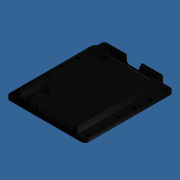
# Autodesk Inventor part: (45-0005) SpartanPi Base Housing
Saved by Autodesk Inventor 2015 (Build 190159000, 159)
## iProperties
Created: 2016-09-21
Part Number: (45-0005) SpartanPi Base Housing
Material: Generic
Document SubType Name: Modeling
Designer: Justin
Density: 1 g/cm^3
Appearance: Smooth - Black
Author: Justin
Autodesk Inventor part; units mm, degrees
ref_plane "YZ Plane" through (0, 0, 0) normal (1, 0, 0) x (0, 1, 0)
ref_plane "XZ Plane" through (0, 0, 0) normal (0, 1, 0) x (-1, 0, 0)
ref_plane "XY Plane" through (0, 0, 0) normal (0, 0, 1) x (1, 0, 0)
sketch "Sketch1" plane through (0, 0, 0) normal (0, 0, 1) x (1, 0, 0)
  line L0 (0, 0) -> (61, 0)
  line L1 (61, 0) -> (61, 90)
  line L2 (61, 90) -> (0, 90)
  line L3 (0, 90) -> (0, 0)
  dimension "d0" = 61
  dimension "d1" = 90
  constraints: 8 end point, 2 parallel, 1 horizontal, 1 perpendicular
  measures "d0" distance of L1.end L2.end
  measures "d1" distance of L0.end L1.end
extrude "Extrusion1" add sketch "Sketch1" along normal blind 10
fillet "Fillet1" radius 3 4 edges at (61, 90, 5) (0, 90, 5) (0, 0, 5) (61, 0, 5)
shell "Shell1" thickness 2 removed faces 1 at (40.6667, 31, 10)
sketch "Sketch8" plane through (0, 0, 10) normal (0, 0, 1) x (1, 0, 0)
  arc A0 (2, 3) -> (3, 2) centre (3, 3) ccw projected
  line L0 (2, 3) -> (2, 87) projected
  arc A1 (3, 88) -> (2, 87) centre (3, 87) ccw projected
  line L1 (3, 88) -> (58, 88) projected
  arc A2 (59, 87) -> (58, 88) centre (58, 87) ccw projected
  line L2 (59, 87) -> (59, 3) projected
  arc A3 (58, 2) -> (59, 3) centre (58, 3) ccw projected
  line L3 (58, 2) -> (3, 2) projected
  line L4 (58, 89.05) -> (3, 89.05)
  arc A4 (3, 89.05) -> (0.95, 87) centre (3, 87) ccw
  line L5 (0.95, 87) -> (0.95, 3)
  arc A5 (0.95, 3) -> (3, 0.95) centre (3, 3) ccw
  line L6 (3, 0.95) -> (58, 0.95)
  arc A6 (58, 0.95) -> (60.05, 3) centre (58, 3) ccw
  line L7 (60.05, 3) -> (60.05, 87)
  arc A7 (60.05, 87) -> (58, 89.05) centre (58, 87) ccw
  point P0 (0, 0)
  dimension "d59" = 1.05
  constraints: 8 end point, 8 point on circle, 4 centre point, 7 other
  measures "d59" distance between parallel lines of L4 L1
extrude "Extrusion8" cut sketch "Sketch8" against normal blind 1.05
sketch "Sketch2" plane through (3, 88, 2) normal (0, 0, 1) x (1, 0, 0)
  line L0 (56, -85) -> (56, -1) projected
  line L1 (55, 0) -> (0, 0) projected
  circle A0 centre (52, -4) radius 3
  circle A1 centre (52, -62) radius 3
  circle A2 centre (3, -4) radius 3
  circle A3 centre (3, -62) radius 3
  point P0 (-3, -88)
  dimension "d6" = 6
  dimension "d7" = 4
  dimension "d8" = 4
  dimension "d11" = 58
  dimension "d14" = 49
  constraints: 4 centre point, 1 horizontal, 1 vertical, 6 other
  measures "d6" diameter of A0
  measures "d7" distance from line of L1 A0.centre
  measures "d8" distance from line of L0 A0.centre
  measures "d11" distance of A0.centre A1.centre
  measures "d14" distance of A0.centre A2.centre
extrude "Extrusion2" add sketch "Sketch2" along normal blind 4
sketch "Sketch3" plane through (6, 26, 6) normal (0, 0, 1) x (1, 0, 0)
  circle A0 centre (0, 0) radius 3 projected
  circle A1 centre (49, 0) radius 3 projected
  circle A2 centre (49, 58) radius 3 projected
  circle A3 centre (0, 58) radius 3 projected
  circle A4 centre (49, 58) radius 1.125
  circle A5 centre (49, 0) radius 1.125
  circle A6 centre (0, 0) radius 1.125
  circle A7 centre (0, 58) radius 1.125
  point P0 (-6, -26)
  dimension "d19" = 2.25
  dimension "d20" = 2.25
  dimension "d21" = 2.25
  dimension "d22" = 2.25
  constraints: 4 centre point, 4 coincident
  measures "d19" diameter of A4
  measures "d20" diameter of A5
  measures "d21" diameter of A6
  measures "d22" diameter of A7
extrude "Extrusion3" cut sketch "Sketch3" against normal blind 10 contours A4 | A5 | A6 | A7
fillet "Fillet2" radius 0.9 8 edges at (2.2929, 2.2929, 2) (30.5, 2, 2) (58.7071, 2.2929, 2) (59, 45, 2) (58.7071, 87.7071, 2) (30.5, 88, 2) (2.2929, 87.7071, 2) (2, 45, 2)
sketch "Sketch9" plane through (3, 0, 0) normal (0, -1, 0) x (1, 0, 0)
  line L0 (0, 10) -> (55, 10) projected
  line L1 (0, 0) -> (0, 10) projected
  line L2 (1.4, 10) -> (18.3, 10)
  line L3 (18.3, 10) -> (18.3, 7.5)
  line L4 (18.3, 7.5) -> (1.4, 7.5)
  line L5 (1.4, 7.5) -> (1.4, 10)
  line L6 (55, 10) -> (0, 10) projected
  line L7 (21.5, 10) -> (35.6, 10)
  line L8 (35.6, 10) -> (35.6, 7.5)
  line L9 (35.6, 7.5) -> (21.5, 7.5)
  line L10 (21.5, 7.5) -> (21.5, 10)
  line L11 (39.5, 10) -> (53.6, 10)
  line L12 (53.6, 10) -> (53.6, 7.5)
  line L13 (53.6, 7.5) -> (39.5, 7.5)
  line L14 (39.5, 7.5) -> (39.5, 10)
  point P0 (-3, 0)
  point P1 (-3, 10)
  point P2 (58, 10)
  dimension "d62" = 16.9
  dimension "d63" = 2.5
  dimension "d64" = 14.1
  dimension "d65" = 2.5
  dimension "d66" = 14.1
  dimension "d67" = 2.5
  dimension "d68" = 3.2
  dimension "d69" = 3.9
  dimension "d70" = 1.4
  constraints: 24 end point, 6 parallel, 3 horizontal, 3 perpendicular, 3 point on line
  measures "d62" distance of L3.end L4.end
  measures "d63" distance of L2.end L3.end
  measures "d64" distance of L8.end L9.end
  measures "d65" distance of L7.end L8.end
  measures "d66" distance of L12.end L13.end
  measures "d67" distance of L11.end L12.end
  measures "d68" distance between parallel lines of L10 L3
  measures "d69" distance between parallel lines of L14 L8
  measures "d70" distance between parallel lines of L1 L5
extrude "Extrusion9" cut sketch "Sketch9" against normal blind 3
sketch "Sketch10" plane through (3, 0, 0) normal (0, -1, 0) x (1, 0, 0)
  line L0 (21.5, 7.5) -> (21.5, 10) projected
  line L1 (0, 10) -> (55, 10) projected
  line L2 (53.6, 10) -> (53.6, 7.5) projected
  line L3 (39.5, 7.5) -> (39.5, 10) projected
  line L4 (0, 10) -> (55, 10) projected
  line L5 (35.6, 10) -> (35.6, 7.5) projected
  line L6 (35.6, 7.5) -> (21.5, 7.5) projected
  line L7 (20.5, 10) -> (36.6, 10)
  line L8 (36.6, 10) -> (36.6, 6.5)
  line L9 (36.6, 6.5) -> (20.5, 6.5)
  line L10 (20.5, 6.5) -> (20.5, 10)
  line L11 (38.5, 10) -> (54.6, 10)
  line L12 (54.6, 10) -> (54.6, 6.5)
  line L13 (54.6, 6.5) -> (38.5, 6.5)
  line L14 (38.5, 6.5) -> (38.5, 10)
  point P0 (-3, 0)
  point P1 (-3, 10)
  point P2 (58, 10)
  dimension "d73" = 1
  dimension "d74" = 1
  dimension "d75" = 1
  dimension "d76" = 1
  dimension "d77" = 1
  constraints: 16 end point, 4 parallel, 3 point on line, 2 horizontal, 2 perpendicular
  measures "d73" distance between parallel lines of L0 L10
  measures "d74" distance between parallel lines of L6 L9
  measures "d75" distance between parallel lines of L8 L5
  measures "d76" distance between parallel lines of L3 L14
  measures "d77" distance between parallel lines of L2 L12
extrude "Extrusion10" cut sketch "Sketch10" against normal blind 0.95
sketch "Sketch11" plane through (0, 3, 0) normal (-1, 0, 0) x (0, 0, 1)
  line L0 (10, 0) -> (10, 84) projected
  line L1 (10, 60.5) -> (7.5, 60.5)
  line L2 (7.5, 60.5) -> (7.5, 44)
  line L3 (7.5, 44) -> (10, 44)
  line L4 (10, 44) -> (10, 60.5)
  line L5 (10, 78.15) -> (6.5, 78.15)
  line L6 (6.5, 78.15) -> (6.5, 69.15)
  line L7 (6.5, 69.15) -> (10, 69.15)
  line L8 (10, 69.15) -> (10, 78.15)
  line L9 (0, -3) -> (10, -3) projected
  dimension "d81" = 16.5
  dimension "d82" = 2.5
  dimension "d83" = 3.5
  dimension "d84" = 9
  dimension "d85" = 8.65
  dimension "d142" = 47
  constraints: 16 end point, 4 parallel, 2 horizontal, 2 perpendicular, 2 point on line
  measures "d81" distance of L1.end L2.end
  measures "d82" distance of L2.end L3.end
  measures "d83" distance of L6.end L7.end
  measures "d84" distance of L5.end L6.end
  measures "d85" distance between parallel lines of L1 L7
  measures "d142" distance between parallel lines of L3 L9
extrude "Extrusion11" cut sketch "Sketch11" against normal blind 3 contours L3 L2 L1 L0
sketch "Sketch12" plane through (0, 3, 0) normal (-1, 0, 0) x (0, 0, 1)
  line L0 (10, 44) -> (7.5, 44) projected
  line L1 (7.5, 44) -> (7.5, 60.5) projected
  line L2 (7.5, 60.5) -> (10, 60.5) projected
  line L3 (10, 84) -> (10, 0) projected
  line L4 (10, 61.5) -> (6.5, 61.5)
  line L5 (6.5, 61.5) -> (6.5, 43)
  line L6 (6.5, 43) -> (10, 43)
  line L7 (10, 43) -> (10, 61.5)
  arc A0 (8.95, 34.0757) -> (8.95, 27.9243) centre (10, 31) ccw projected
  point P0 (0, -3)
  point P1 (10, 87)
  point P2 (10, -3)
  dimension "d93" = 1
  dimension "d94" = 1
  dimension "d95" = 1
  constraints: 8 end point, 2 parallel, 1 horizontal, 1 perpendicular, 1 point on line
  measures "d93" distance between parallel lines of L2 L4
  measures "d94" distance between parallel lines of L1 L5
  measures "d95" distance between parallel lines of L0 L6
extrude "Extrusion12" cut sketch "Sketch12" against normal blind 0.95
fillet "Fillet3" radius 0.5 6 edges at (23.5, 0, 8.25) (31.55, 0, 6.5) (39.6, 0, 8.25) (41.5, 0, 8.25) (49.55, 0, 6.5) (57.6, 0, 8.25)
sketch "Sketch13" plane through (3, 90, 0) normal (0, 1, 0) x (1, 0, 0)
  line L0 (55, 0) -> (55, -10) projected
  line L1 (0, -10) -> (55, -10) projected
  line L2 (34.25, -10) -> (20.75, -10)
  line L3 (20.75, -10) -> (20.75, -3)
  line L4 (20.75, -3) -> (34.25, -3)
  line L5 (34.25, -3) -> (34.25, -10)
  point P0 (-3, 0)
  dimension "d101" = 7
  dimension "d102" = 13.5
  dimension "d103" = 20.75
  constraints: 8 end point, 2 parallel, 1 horizontal, 1 perpendicular, 1 point on line
  measures "d101" distance of L2.end L3.end
  measures "d102" distance of L3.end L4.end
  measures "d103" distance between parallel lines of L0 L5
extrude "Extrusion13" cut sketch "Sketch13" against normal blind 3
fillet "Fillet5" radius 2 2 edges at (37.25, 89, 3) (23.75, 89, 3)
sketch "Sketch4" plane through (0, 0, 0) normal (0, 0, -1) x (-1, 0, 0)
  arc A0 (-61, 3) -> (-58, 0) centre (-58, 3) ccw projected
  arc A1 (-3, 0) -> (0, 3) centre (-3, 3) ccw projected
  line L0 (0, 90) -> (0, 0) projected
  arc A2 (0, 87) -> (-3, 90) centre (-3, 87) ccw projected
  arc A3 (-58, 90) -> (-61, 87) centre (-58, 87) ccw projected
  line L1 (-61, 0) -> (-61, 90) projected
  line L2 (-3, 0) -> (5.5, 0)
  line L3 (9.5, 4) -> (9.5, 86)
  line L4 (5.5, 90) -> (-3, 90)
  line L5 (-58, 90) -> (-66.5, 90)
  line L6 (-70.5, 86) -> (-70.5, 4)
  line L7 (-66.5, 0) -> (-58, 0)
  arc A4 (-61, 3) -> (-58, 0) centre (-58, 3) ccw projected
  arc A5 (5.5, 0) -> (9.5, 4) centre (5.5, 4) ccw
  arc A6 (-70.5, 4) -> (-66.5, 0) centre (-66.5, 4) ccw
  arc A7 (-66.5, 90) -> (-70.5, 86) centre (-66.5, 86) ccw
  arc A8 (9.5, 86) -> (5.5, 90) centre (5.5, 86) ccw
  point P0 (-70.5, 90)
  point P1 (-70.5, 0)
  dimension "d26" = 9.5
  dimension "d27" = 9.5
  dimension "d28" = 4
  constraints: 12 end point, 12 tangent, 8 point on circle, 6 point on line, 4 centre point, 4 perpendicular, 3 equal radius, 1 horizontal
  measures "d26" distance between parallel lines of L0 L3
  measures "d27" distance between parallel lines of L1 L6
  measures "d28" radius of A5
extrude "Extrusion4" add sketch "Sketch4" against normal blind 3
sketch "Sketch14" plane through (37.25, 90, 10) normal (0, 1, 0) x (1, 0, 0)
  line L0 (-13.5, 0) -> (-13.5, 5) projected
  arc A0 (-11.5, 7) -> (-13.5, 5) centre (-11.5, 5) ccw projected
  line L1 (-11.5, 7) -> (-2, 7) projected
  arc A1 (0, 5) -> (-2, 7) centre (-2, 5) ccw projected
  line L2 (0, 5) -> (0, 0) projected
  line L3 (20.75, 0) -> (0, 0) projected
  line L4 (-13.5, 0) -> (-34.25, 0) projected
  line L5 (1, 0) -> (1, 5)
  arc A2 (1, 5) -> (-2, 8) centre (-2, 5) ccw
  line L6 (-2, 8) -> (-11.5, 8)
  arc A3 (-11.5, 8) -> (-14.5, 5) centre (-11.5, 5) ccw
  line L7 (-14.5, 5) -> (-14.5, 0)
  point P0 (-37.25, 10)
  dimension "d119" = 1
  constraints: 6 end point, 4 point on circle, 2 centre point, 2 point on line, 4 other
  measures "d119" distance between parallel lines of L2 L5
extrude "Extrusion14" cut sketch "Sketch14" against normal blind 0.95
sketch "Sketch5" plane through (0, 0, 0) normal (0, 0, -1) x (-1, 0, 0)
  line L0 (0, 0) -> (-66.5, 0) projected
  line L1 (9.5, 4) -> (9.5, 86) projected
  circle A0 centre (5.5, 5) radius 2.1
  point P0 (-3, 0)
  point P1 (-58, 0)
  point P2 (-61, 0)
  dimension "d31" = 4.2
  dimension "d32" = 4
  dimension "d33" = 5
  constraints: 1 centre point
  measures "d31" diameter of A0
  measures "d32" distance from line of L1 A0.centre
  measures "d33" distance from line of L0 A0.centre
extrude "Extrusion5" cut sketch "Sketch5" against normal blind 3
pattern_linear "Rectangular Pattern1" count 6 spacing 16 along (0, 1, 0) count 2 spacing 72 along (1, 0, 0) of "Extrusion5"
sketch "Sketch15" plane through (2, 3, 2.9) normal (1, 0, 0) x (0, 0, -1)
  line L0 (-6.05, 60.5) -> (-4.6, 60.5) projected
  line L1 (-7.1, 61.5) -> (-7.1, 84) projected
  line L2 (-7.1, 68.15) -> (-3.6, 68.15)
  line L3 (-3.6, 68.15) -> (-3.6, 79.15)
  line L4 (-3.6, 79.15) -> (-7.1, 79.15)
  line L5 (-7.1, 79.15) -> (-7.1, 68.15)
  point P0 (2.9, -3)
  dimension "d123" = 11
  dimension "d124" = 3.5
  dimension "d125" = 7.65
  constraints: 8 end point, 2 parallel, 1 horizontal, 1 perpendicular, 1 point on line
  measures "d123" distance of L2.end L3.end
  measures "d124" distance of L3.end L4.end
  measures "d125" distance between parallel lines of L0 L2
extrude "Extrusion15" cut sketch "Sketch15" against normal blind 1.05
chamfer "Chamfer5" distance 0.95 angle 45 3 edges at (0, 64.5, 8.25) (0, 55.25, 6.5) (0, 46, 8.25)
sketch "Sketch17" plane through (37.25, 89.05, 10) normal (0, 1, 0) x (1, 0, 0)
  line L0 (0, 1.05) -> (1, 1.05) projected
  line L1 (1, 5) -> (1, 1.05) projected
  line L2 (-14.5, 1.05) -> (-14.5, 5) projected
  line L3 (-14.5, 1.05) -> (-13.5, 1.05) projected
  line L4 (-13.5, 5) -> (-13.5, 1.05) projected
  line L5 (0, 1.05) -> (0, 5) projected
  line L6 (0, 3) -> (0.95, 3) projected
  line L7 (-14.45, 3) -> (-13.5, 3) projected
  line L8 (0, 3) -> (1, 3)
  line L9 (1, 3) -> (1, 3.05)
  line L10 (1, 3.05) -> (0, 3.05)
  line L11 (0, 3.05) -> (0, 3)
  line L12 (-13.5, 3) -> (-14.5, 3)
  line L13 (-14.5, 3) -> (-14.5, 3.05)
  line L14 (-14.5, 3.05) -> (-13.5, 3.05)
  line L15 (-13.5, 3.05) -> (-13.5, 3)
  point P0 (-14.5, 5)
  point P1 (-37.25, 10)
  dimension "d132" = 1
  dimension "d133" = 0.05
  dimension "d134" = 1
  dimension "d135" = 0.05
  constraints: 16 end point, 4 parallel, 2 horizontal, 2 perpendicular, 2 other
  measures "d132" distance of L10.end L9.end
  measures "d133" distance of L9.end L8.end
  measures "d134" distance of L13.end L14.end
  measures "d135" distance of L12.end L13.end
extrude "Extrusion16" cut sketch "Sketch17" against normal blind 10
sketch "Sketch19" plane through (0, 3, 3) normal (-1, 0, 0) x (0, 0, 1)
  line L0 (7, 42.05) -> (7, 0) projected
  circle A0 centre (7.3, 30.7) radius 3.5
  line L1 (0, -3) -> (7, -3) projected
  point P0 (-3, -3)
  dimension "d143" = 7
  dimension "d144" = 0.3
  dimension "d145" = 33.7
  constraints: 1 centre point
  measures "d143" diameter of A0
  measures "d144" distance from line of L0 A0.centre
  measures "d145" distance from line of L1 A0.centre
extrude "Extrusion17" cut sketch "Sketch19" against normal blind 10
sketch "Sketch20" plane through (0, 0, 0) normal (0, 0, -1) x (-1, 0, 0)
  line L0 (-51, 32.5) -> (-10, 32.5)
  line L1 (-8, 34.5) -> (-8, 75.5)
  line L2 (-10, 77.5) -> (-51, 77.5)
  line L3 (-53, 75.5) -> (-53, 34.5)
  arc A0 (-53, 34.5) -> (-51, 32.5) centre (-51, 34.5) ccw
  arc A1 (-51, 77.5) -> (-53, 75.5) centre (-51, 75.5) ccw
  arc A2 (-8, 75.5) -> (-10, 77.5) centre (-10, 75.5) ccw
  arc A3 (-10, 32.5) -> (-8, 34.5) centre (-10, 34.5) ccw
  circle A4 centre (-6, 26) radius 1.125 projected
  circle A5 centre (-55, 26) radius 1.125 projected
  point P0 (0, 0)
  point P1 (-53, 32.5)
  point P2 (-8, 77.5)
  point P3 (-8, 32.5)
  dimension "d148" = 45
  dimension "d149" = 45
  dimension "d152" = 2
  dimension "d158" = 2
  dimension "d159" = 6.5
  constraints: 8 end point, 8 point on circle, 8 tangent, 6 point on line, 4 centre point, 3 equal radius, 2 parallel, 1 horizontal, 1 perpendicular
  measures "d148" distance of point (-53, 32.5) point (-8, 32.5)
  measures "d149" distance of point (-8, 32.5) point (-8, 77.5)
  measures "d152" radius of A0
  measures "d158" distance from line of L3 A5.centre
  measures "d159" distance from line of A5.centre L0
extrude "Extrusion18" cut sketch "Sketch20" against normal blind 0.25 contours A0 L3 A1 L2 A2 L1 A3 L0
chamfer "Chamfer7" distance 0.5 angle 45 1 edges at (0, 33.7, 6.8)
sketch "Sketch21" plane through (3, 2.9, 2) normal (0, 0, 1) x (1, 0, 0)
  circle A0 centre (3, 23.1) radius 3 projected
  circle A1 centre (52, 23.1) radius 3 projected
  circle A2 centre (52, 81.1) radius 3 projected
  circle A3 centre (3, 81.1) radius 3 projected
  circle A4 centre (3, 81.1) radius 4
  circle A5 centre (52, 81.1) radius 3 projected
  circle A6 centre (52, 81.1) radius 4
  circle A7 centre (3, 23.1) radius 4
  circle A8 centre (52, 23.1) radius 4
  point P0 (-3, -2.9)
  dimension "d160" = 8
  dimension "d161" = 8
  dimension "d162" = 8
  dimension "d163" = 8
  constraints: 4 centre point, 4 coincident
  measures "d160" diameter of A4
  measures "d161" diameter of A6
  measures "d162" diameter of A7
  measures "d163" diameter of A8
extrude "Extrusion19" add sketch "Sketch21" along normal blind 3
sketch "Sketch22" plane through (0, 0, 0) normal (0, 0, -1) x (-1, 0, 0)
  circle A0 centre (-55, 84) radius 1.125 projected
  circle A1 centre (-6, 26) radius 1.125 projected
  circle A2 centre (-55, 26) radius 1.125 projected
  circle A3 centre (-6, 84) radius 1.125 projected
  circle A4 centre (-55, 26) radius 2.5
  circle A5 centre (-55, 84) radius 1.125 projected
  circle A6 centre (-55, 84) radius 2.5
  circle A7 centre (-6, 26) radius 2.5
  circle A8 centre (-6, 84) radius 2.5
  point P0 (0, 0)
  dimension "d166" = 5
  dimension "d167" = 5
  dimension "d168" = 5
  dimension "d169" = 5
  constraints: 4 centre point, 4 coincident
  measures "d166" diameter of A4
  measures "d167" diameter of A6
  measures "d168" diameter of A7
  measures "d169" diameter of A8
extrude "Extrusion20" cut sketch "Sketch22" against normal blind 4
fillet "Fillet7" radius 1 4 edges at (52, 84, 5) (52, 26, 5) (3, 26, 5) (3, 84, 5)
fillet "Fillet8" radius 0.4 8 edges at (8.5, 84, 4) (57.5, 84, 4) (8.5, 26, 4) (57.5, 26, 4) (57.5, 26, 0) (8.5, 26, 0) (8.5, 84, 0) (57.5, 84, 0)
body "Solid1"
